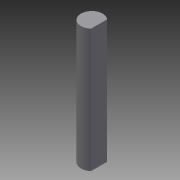
# Autodesk Inventor part: DMJ_arm
Saved by Autodesk Inventor 2015 SP1 (Build 190203100, 203)
## iProperties
Created: 2016-02-03
Part Number: DMJ_arm
Material: Generic
Document SubType Name: Modeling
Designer: guillemd
Density: 1 g/cm^3
Appearance: Default
Author: guillemd
Autodesk Inventor part; units mm, degrees
ref_plane "YZ Plane" through (0, 0, 0) normal (1, 0, 0) x (0, 1, 0)
ref_plane "XZ Plane" through (0, 0, 0) normal (0, 1, 0) x (-1, 0, 0)
ref_plane "XY Plane" through (0, 0, 0) normal (0, 0, 1) x (1, 0, 0)
sketch "Sketch1" plane through (0, 0, 0) normal (0, 1, 0) x (-1, 0, 0)
  arc A0 (0, -56.7961) -> (0, 56.7961) centre (50.8, 0) ccw
  line L0 (0, -106.68) -> (0, 106.68) projected
  line L1 (152.4, 0) -> (-25.4, 0) projected
  line L2 (0, 56.7961) -> (0, -56.7961)
  point P0 (0, 0)
  point P1 (127, 0)
  dimension "d0" = 76.2
  dimension "d1" = 127
  constraints: 3 point on circle, 3 point on line, 2 end point, 1 centre point, 1 collinear
  measures "d0" radius of A0
  measures "d1" distance from line of L0 point (127, 0)
extrude "Extrusion1" add sketch "Sketch1" along normal blind 866.14
body "Solid1"
